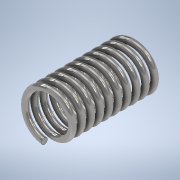
# Autodesk Inventor part: mola
Saved by Autodesk Inventor 2022.2 (Build 262287010, 287A)
## iProperties
Created: 2022-05-04
Part Number: mola
Material: Steel, Mild
Document SubType Name: Modeling
Designer: Korch
Density: 7.85 g/cm^3
Appearance: Semi-Polished
Author: Korch
Autodesk Inventor part; units mm, degrees
ref_plane "YZ Plane" through (0, 0, 0) normal (1, 0, 0) x (0, 1, 0)
ref_plane "XZ Plane" through (0, 0, 0) normal (0, 1, 0) x (-1, 0, 0)
sketch "Sketch4" plane through (0, 0, 0) normal (1, 0, 0) x (0, 1, 0)
  line L0 (0, 0) -> (0, 15)
  line L1 (0, 0) -> (-3.5, 0)
  circle A0 centre (-3.5, 0) radius 0.5
  dimension "d26" = 15
  dimension "d27" = 3.5
  dimension "d28" = 1
  constraints: 4 end point, 1 centre point, 1 coincident, 1 horizontal, 1 vertical
  measures "d26" distance of L0.start L0.end
  measures "d27" distance of L0.start L1.end
  measures "d28" diameter of A0
coil "Coil3" sketch "Sketch4" operation add axis through (0, 0, 0) along (0, 0, 1) pitch 1.5 turns 10 hand right
ref_plane "Work Plane3" through (0, 0, 15) normal (0, 0, 1) x (1, 0, 0)
body "Solid3"
